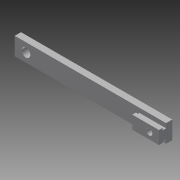
# Autodesk Inventor part: Piece One-Diagonal Piece
Saved by Autodesk Inventor 2013 (Build 170138000, 138)
## iProperties
Created: 2014-05-23
Part Number: Piece One-Diagonal Piece
Material: Steel
Document SubType Name: Modeling
Designer: nojessen
Density: 1 g/cm^3
Author: nojessen
Autodesk Inventor part; units mm, degrees
ref_plane "YZ Plane" through (0, 0, 0) normal (1, 0, 0) x (0, 1, 0)
ref_plane "XZ Plane" through (0, 0, 0) normal (0, 1, 0) x (-1, 0, 0)
ref_plane "XY Plane" through (0, 0, 0) normal (0, 0, 1) x (1, 0, 0)
sketch "Sketch1" plane through (0, 0, 0) normal (0, 0, 1) x (1, 0, 0)
  line L0 (0, 0) -> (215.9, 0)
  line L1 (215.9, 0) -> (215.9, 25.4)
  line L2 (215.9, 25.4) -> (0, 25.4)
  line L3 (0, 25.4) -> (0, 0)
  dimension "d0" = 215.9
  dimension "d1" = 25.4
  constraints: 8 end point, 2 parallel, 1 horizontal, 1 perpendicular
  measures "d0" distance of L2.end L1.end
  measures "d1" distance of L1.end L0.end
extrude "Extrusion1" add sketch "Sketch1" along normal blind 8.89
sketch "Sketch2" plane through (0, 0, 8.89) normal (0, 0, 1) x (1, 0, 0)
  line L0 (0, 0) -> (215.9, 0) projected
  line L1 (215.9, 0) -> (215.9, 25.4) projected
  line L2 (215.9, 25.4) -> (177.8, 25.4)
  line L3 (177.8, 25.4) -> (177.8, 0)
  line L4 (177.8, 0) -> (215.9, 0)
  line L5 (215.9, 0) -> (215.9, 25.4)
  line L6 (215.9, 25.4) -> (177.8, 25.4)
  line L7 (177.8, 25.4) -> (177.8, 12.7)
  line L8 (177.8, 12.7) -> (215.9, 12.7)
  line L9 (215.9, 12.7) -> (215.9, 25.4)
  line L10 (215.9, 25.4) -> (177.8, 25.4)
  line L11 (177.8, 25.4) -> (177.8, 19.05)
  line L12 (177.8, 19.05) -> (215.9, 19.05)
  line L13 (215.9, 19.05) -> (215.9, 25.4)
  line L14 (215.9, 0) -> (177.8, 0)
  line L15 (177.8, 0) -> (177.8, 6.35)
  line L16 (177.8, 6.35) -> (215.9, 6.35)
  line L17 (215.9, 6.35) -> (215.9, 0)
  dimension "d4" = 6.35
  dimension "d5" = 38.1
  constraints: 32 end point, 8 parallel, 4 horizontal, 4 perpendicular, 2 midpoint, 2 point on line
  measures "d4" distance of L14.end L15.end
  measures "d5" distance between parallel lines of L13 L11
extrude "Extrusion2" add sketch "Sketch2" along normal blind 5.08 contours L3 L8 L1 L16 | L3 L12 L1 L8
sketch "Sketch3" plane through (0, 0, 13.97) normal (0, 0, 1) x (1, 0, 0)
  line L0 (215.9, 19.05) -> (177.8, 19.05) projected
  line L1 (177.8, 19.05) -> (177.8, 6.35) projected
  line L2 (177.8, 6.35) -> (215.9, 6.35)
  line L3 (215.9, 6.35) -> (215.9, 19.05)
  line L4 (215.9, 19.05) -> (177.8, 19.05)
  line L5 (177.8, 19.05) -> (177.8, 6.35)
  line L6 (215.9, 19.05) -> (177.8, 19.05)
  line L7 (177.8, 19.05) -> (177.8, 21.971)
  line L8 (177.8, 21.971) -> (215.9, 21.971)
  line L9 (215.9, 21.971) -> (215.9, 19.05)
  line L10 (215.9, 6.35) -> (177.8, 6.35)
  line L11 (177.8, 6.35) -> (177.8, 3.429)
  line L12 (177.8, 3.429) -> (215.9, 3.429)
  line L13 (215.9, 3.429) -> (215.9, 6.35)
  point P0 (0, 0)
  dimension "d8" = 2.921
  dimension "d9" = 2.921
  constraints: 24 end point, 6 parallel, 3 horizontal, 3 perpendicular
  measures "d8" distance of L6.end L7.end
  measures "d9" distance of L11.end L10.end
extrude "Extrusion3" add sketch "Sketch3" along normal blind 5.08
sketch "Sketch4" plane through (0, 0, 0) normal (0, 0, -1) x (-1, 0, 0)
  circle A0 centre (-202.0681, 12.7) radius 4.445
  dimension "d12" = 8.89
  constraints: 1 centre point
  measures "d12" diameter of A0
extrude "Extrusion4" cut sketch "Sketch4" against normal blind 127
sketch "Sketch5" plane through (0, 0, 8.89) normal (0, 0, 1) x (1, 0, 0)
  circle A0 centre (15.8377, 12.7) radius 6.35
  dimension "d17" = 12.7
  constraints: 1 centre point
  measures "d17" diameter of A0
extrude "Extrusion5" cut sketch "Sketch5" against normal blind 25.4
body "Solid1"
